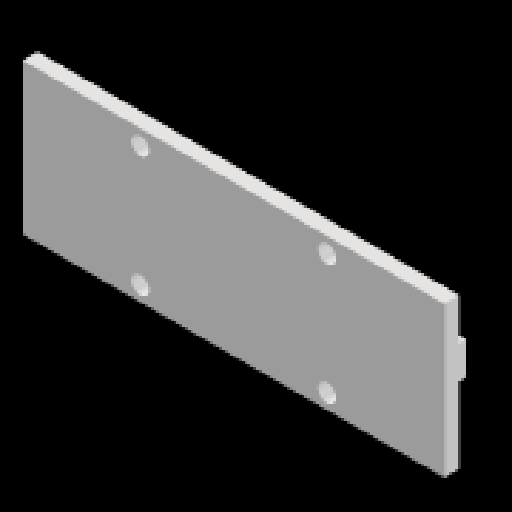
# Autodesk Inventor part: CombineTestBase
Saved by Autodesk Inventor 2025 (Build 290162000, 162)
## iProperties
Created: 2025-01-20
Part Number: CombineTestBase
Material: Generic
Document SubType Name: Modeling
Designer: Trevor
Density: 1 g/cm^3
Appearance: Default
Author: Trevor
Autodesk Inventor part; units mm, degrees
ref_plane "YZ Plane" through (0, 0, 0) normal (1, 0, 0) x (0, 1, 0)
ref_plane "XZ Plane" through (0, 0, 0) normal (0, 1, 0) x (-1, 0, 0)
ref_plane "XY Plane" through (0, 0, 0) normal (0, 0, 1) x (1, 0, 0)
sketch "Sketch1" plane through (0, 0, 0) normal (0, 0, 1) x (1, 0, 0)
  line L0 (65, 8) -> (65, -5) projected
  line L1 (-5, -5) -> (-5, 8) projected
  line L2 (-5, 8) -> (65, 8) projected
  line L3 (65, 8) -> (65, -5) projected
  line L4 (65, -5) -> (-5, -5) projected
  line L5 (-5, 15) -> (65, 15)
  line L6 (65, 15) -> (65, -10)
  line L7 (65, -10) -> (-5, -10)
  line L8 (-5, -10) -> (-5, 15)
  line L9 (-5, 15) -> (65, -10) construction
  line L10 (65, 15) -> (-5, -10) construction
  point P0 (0, 0)
  point P1 (30, 2.5)
  dimension "d0" = 25
  constraints: 12 end point, 2 midpoint, 2 parallel, 1 perpendicular
  measures "d0" distance of L5.end L6.end
extrude "Extrusion1" add sketch "Sketch1" along normal blind 2.5
sketch "Sketch2" plane through (0, 0, 0) normal (0, 0, -1) x (-1, 0, 0)
  line L0 (-60, 0) -> (0, 0) projected
  line L1 (0, 0) -> (0, 3) projected
  line L2 (-60, 3) -> (0, 3) projected
  line L3 (-60, 0) -> (-60, 3) projected
  line L4 (0.2, -0.2) -> (-60.2, -0.2)
  line L5 (-60.2, -0.2) -> (-60.2, 3.2)
  line L6 (-60.2, 3.2) -> (0.2, 3.2)
  line L7 (0.2, 3.2) -> (0.2, -0.2)
  line L8 (-61.2, -1.2) -> (1.2, -1.2)
  line L9 (1.2, -1.2) -> (1.2, 4.2)
  line L10 (1.2, 4.2) -> (-61.2, 4.2)
  line L11 (-61.2, 4.2) -> (-61.2, -1.2)
  dimension "d3" = 0.2
  dimension "d4" = 1
  constraints: 16 end point, 6 other
  measures "d3" distance between parallel lines of L0 L4
  measures "d4" distance between parallel lines of L4 L8
extrude "Extrusion2" add sketch "Sketch2" along normal blind 5 contours L11 L10 L9 L8
fillet "Fillet1" radius 2 4 edges at (30, -1.2, 0) (-1.2, 1.5, 0) (30, 4.2, 0) (61.2, 1.5, 0)
sketch "Sketch3" plane through (0, 0, 0) normal (0, 0, -1) x (-1, 0, 0)
  line L0 (-65, -9.278) -> (-65, -5)
  line L1 (-47.2, 0) -> (-43.8, 0) projected
  line L2 (-45.5, 0) -> (-45.5, -10) construction
  line L3 (-16.2, 0) -> (-12.8, 0) projected
  line L4 (-14.5, 0) -> (-14.5, -7.5)
  circle A0 centre (-14.5, -7.5) radius 1.5
  line L5 (5, -10) -> (-65, -10) construction
  circle A1 centre (-14.5, -7.5) radius 1.5
  line L6 (-65, 2.5) -> (5, 2.5) construction
  line L7 (-65, -10) -> (-65, -5)
  line L8 (-65, -10) -> (-65, 15) projected
  line L9 (-65, -7.5) -> (5, -7.5) construction
  line L10 (5, 15) -> (5, -10) construction
  circle A2 centre (-45.5, -7.5) radius 1.5
  circle A3 centre (-14.5, 12.5) radius 1.5
  circle A4 centre (-45.5, 12.5) radius 1.5
  point P0 (0, 0)
  dimension "d11" = 3
  dimension "d28" = 3
  constraints: 12 end point, 5 centre point, 4 point on line, 3 midpoint, 2 symmetric about line, 2 vertical, 1 coincident, 1 collinear, 1 perpendicular, 2 other
  measures "d11" diameter of A0
  measures "d28" diameter of A2
extrude "Extrusion3" cut sketch "Sketch3" against normal up to surface (2.5 mm away)
body "Solid1"
